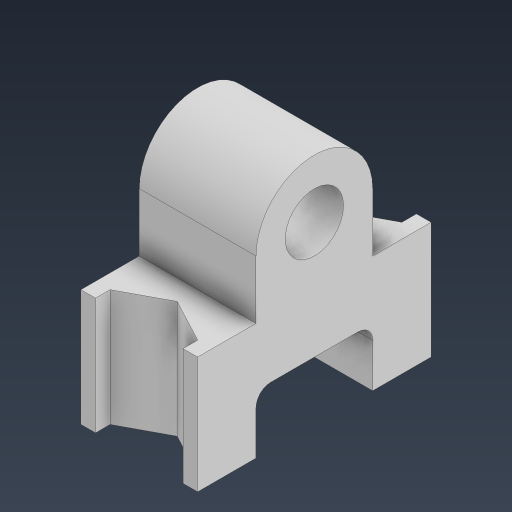
# Autodesk Inventor part: 3D Model
Saved by Autodesk Inventor 2024 (Build 280153000, 153)
## iProperties
Created: 2024-03-05
Part Number: 3D Model
Material: Genérico
Document SubType Name: Modeling
Designer: Administrator
Density: 1 g/cm^3
Appearance: Padrão
Author: Administrator
Autodesk Inventor part; units mm, degrees
ref_plane "YZ Plane" through (0, 0, 0) normal (1, 0, 0) x (0, 1, 0)
ref_plane "XZ Plane" through (0, 0, 0) normal (0, 1, 0) x (-1, 0, 0)
ref_plane "XY Plane" through (0, 0, 0) normal (0, 0, 1) x (1, 0, 0)
sketch "Esboço1" plane through (0, 0, 0) normal (0, 1, 0) x (-1, 0, 0)
  line L0 (20, -40) -> (-20, -40)
  line L1 (-20, -40) -> (-20, 40)
  line L2 (-20, 40) -> (20, 40)
  line L3 (20, 40) -> (20, -40)
  line L4 (20, -40) -> (-20, 40) construction
  line L5 (-20, -40) -> (20, 40) construction
  point P0 (0, 0)
  dimension "d0" = 40
  dimension "d1" = 80
  constraints: 12 end point, 2 midpoint, 2 parallel, 1 horizontal, 1 perpendicular
  measures "d0" distance of L1.end L2.end
  measures "d1" distance of L0.end L1.end
extrude "Extrusão1" add sketch "Esboço1" along normal blind 80
sketch "Esboço2" plane through (20, 0, 40) normal (1, 0, 0) x (0, 0, -1)
  line L0 (0, 80) -> (20, 80)
  line L1 (20, 80) -> (20, 40)
  line L2 (20, 40) -> (0, 40)
  line L3 (0, 40) -> (0, 80)
  line L4 (80, 80) -> (60, 80)
  line L5 (60, 80) -> (60, 40)
  line L6 (60, 40) -> (80, 40)
  line L7 (80, 40) -> (80, 80)
  line L8 (0, 0) -> (80, 0) projected
  point P0 (40, 0)
  dimension "d4" = 20
  dimension "d5" = 20
  dimension "d6" = 40
  constraints: 16 end point, 4 parallel, 2 horizontal, 2 perpendicular, 2 point on line, 1 coincident
  measures "d4" distance of L1.end L2.end
  measures "d5" distance of L5.end L6.end
  measures "d6" distance between parallel lines of L8 L2
extrude "Extrusão2" cut sketch "Esboço2" against normal through all contours L0 L1 L2 L3
extrude "Extrusão3" cut sketch "Esboço2" against normal through all contours L7 L6 L5 L4
fillet "Arredondamento1" radius 20 2 edges at (0, 80, 20) (0, 80, -20)
sketch "Esboço3" plane through (20, 0, 40) normal (1, 0, 0) x (0, 0, -1)
  arc A0 (60, 60) -> (20, 60) centre (40, 60) ccw projected
  point P0 (40, 0)
  constraints: 1 coincident
hole "Furo1" at (20, 60, 0) direction (-1, 0, 0) diameter 20 end through all
sketch "Esboço4" plane through (20, 40, 40) normal (0, 1, 0) x (1, 0, 0)
  line L0 (-35, 0) -> (-35, 5)
  line L1 (-35, 5) -> (-20, 13)
  line L2 (-20, 13) -> (-5, 5)
  line L3 (-5, 5) -> (-5, 0)
  line L4 (-40, 0) -> (-40, 20) projected
  line L5 (0, 0) -> (-40, 0) projected
  point P0 (-20, 40)
  dimension "d19" = 5
  dimension "d20" = 30
  dimension "d21" = 20
  dimension "d22" = 13
  dimension "d23" = 5
  constraints: 8 end point, 2 parallel, 2 point on line, 1 vertical
  measures "d19" distance between parallel lines of L4 L0
  measures "d20" distance between parallel lines of L0 L3
  measures "d21" distance from line of L4 L1.end
  measures "d22" distance from line of L1.end L5
  measures "d23" distance of L0.start L0.end
extrude "Extrusão4" cut sketch "Esboço4" against normal through all
mirror "Espelhar1" about plane through (0, 0, 0) normal (0, 0, 1) of "Extrusão4"
sketch "Esboço6" plane through (20, 0, 40) normal (1, 0, 0) x (0, 0, -1)
  line L0 (20, 20) -> (60, 20)
  line L1 (60, 20) -> (60, 0)
  line L2 (60, 0) -> (20, 0)
  line L3 (20, 0) -> (20, 20)
  line L4 (0, 0) -> (80, 0) projected
  point P0 (40, 0)
  point P1 (40, 0)
  dimension "d26" = 40
  dimension "d27" = 20
  constraints: 8 end point, 2 midpoint, 2 parallel, 1 horizontal, 1 perpendicular
  measures "d26" distance of L1.end L2.end
  measures "d27" distance between parallel lines of L2 L0
extrude "Extrusão5" cut sketch "Esboço6" against normal through all
fillet "Arredondamento2" radius 5 2 edges at (0, 20, -20) (0, 20, 20)
